Autodesk Inventor part; units mm, degrees
(part 2 of 2)
sketch "Sketch8" plane through (0, 0, 6.35) normal (0, 0, 1) x (1, 0, 0)
  line L0 (104.7603, 19.05) -> (104.7603, 12.7) projected
  line L1 (104.7603, 12.7) -> (59.5313, 12.7) projected
  line L2 (59.5313, 12.7) -> (59.5312, -36.7665) projected
  line L3 (59.5312, -36.7665) -> (65.8813, -36.7665) projected
  line L4 (65.8813, -36.7665) -> (65.8813, -43.1165) projected
  line L5 (65.8813, -43.1165) -> (72.2313, -43.1165) projected
  line L6 (72.2313, -43.1165) -> (72.2313, -36.7665) projected
  line L7 (72.2313, -36.7665) -> (78.5813, -36.7665) projected
  line L8 (78.5813, -36.7665) -> (78.5813, -43.1165) projected
  line L9 (78.5813, -43.1165) -> (84.9313, -43.1165) projected
  line L10 (84.9313, -43.1165) -> (84.9313, -36.7665) projected
  line L11 (84.9313, -36.7665) -> (91.2812, -36.7665) projected
  line L12 (91.2812, -36.7665) -> (91.2812, -43.1165) projected
  line L13 (91.2812, -43.1165) -> (97.6313, -43.1165) projected
  line L14 (97.6313, -43.1165) -> (97.6313, -36.7665) projected
  line L15 (97.6313, -36.7665) -> (103.9813, -36.7665) projected
  line L16 (103.9813, -36.7665) -> (103.9813, -43.1165) projected
  line L17 (103.9813, -43.1165) -> (110.3313, -43.1165) projected
  line L18 (110.3313, -43.1165) -> (110.3313, -36.7665) projected
  line L19 (110.3313, -36.7665) -> (116.6813, -36.7665) projected
  line L20 (116.6813, -36.7665) -> (116.6813, -43.1165) projected
  line L21 (116.6813, -43.1165) -> (123.0313, -43.1165) projected
  line L22 (123.0313, -43.1165) -> (123.0313, -36.7665) projected
  line L23 (123.0313, -36.7665) -> (129.3812, -36.7665) projected
  line L24 (129.3812, -36.7665) -> (129.3812, -43.1165) projected
  line L25 (129.3812, -43.1165) -> (135.7313, -43.1165) projected
  line L26 (135.7313, -43.1165) -> (135.7313, -36.7665) projected
  line L27 (135.7313, -36.7665) -> (142.8603, -36.7665) projected
  line L28 (142.8603, -36.7665) -> (142.8603, -43.1165) projected
  arc A0 (142.8603, -43.1165) -> (143.3542, -41.4448) centre (0, 0) ccw projected
  arc A1 (143.3542, -41.4448) -> (149.3949, -41.0801) centre (144.1598, -4.5833) ccw projected
  arc A2 (149.3949, -41.0801) -> (149.9198, -39.121) centre (0, 0) ccw projected
  arc A3 (149.9198, -39.121) -> (144.8708, -35.7848) centre (127.1377, -68.1106) ccw projected
  arc A4 (144.8708, -35.7848) -> (145.3268, -33.8855) centre (0, 0) ccw projected
  arc A5 (145.3268, -33.8855) -> (151.3401, -33.2051) centre (144.2021, 2.9677) ccw projected
  arc A6 (151.3401, -33.2051) -> (151.7618, -31.2212) centre (0, 0) ccw projected
  arc A7 (151.7618, -31.2212) -> (146.5451, -28.1538) centre (130.5281, -61.3634) ccw projected
  arc A8 (146.5451, -28.1538) -> (146.9011, -26.2332) centre (0, 0) ccw projected
  arc A9 (146.9011, -26.2332) -> (152.8705, -25.239) centre (143.8491, 10.5106) ccw projected
  arc A10 (152.8705, -25.239) -> (153.1878, -23.2358) centre (0, 0) ccw projected
  arc A11 (153.1878, -23.2358) -> (147.8177, -20.4457) centre (133.5607, -54.448) ccw projected
  arc A12 (147.8177, -20.4457) -> (148.0727, -18.509) centre (0, 0) ccw projected
  arc A13 (148.0727, -18.509) -> (153.9819, -17.2038) centre (143.1019, 18.0247) ccw projected
  arc A14 (153.9819, -17.2038) -> (154.1939, -15.1868) centre (0, 0) ccw projected
  arc A15 (154.1939, -15.1868) -> (148.6852, -12.6815) centre (136.2272, -47.3834) ccw projected
  arc A16 (148.6852, -12.6815) -> (148.8384, -10.7342) centre (0, 0) ccw projected
  arc A17 (148.8384, -10.7342) -> (154.6713, -9.1214) centre (141.9624, 25.4894) ccw projected
  arc A18 (154.6713, -9.1214) -> (154.7774, -7.0961) centre (0, 0) ccw projected
  arc A19 (154.7774, -7.0961) -> (149.1451, -4.8825) centre (138.5204, -40.1889) ccw projected
  arc A20 (149.1451, -4.8825) -> (149.1962, -2.9298) centre (0, 0) ccw projected
  arc A21 (149.1962, -2.9298) -> (154.9367, -1.0141) centre (140.4339, 32.8842) ccw projected
  arc A22 (154.9367, -1.0141) -> (154.9367, 1.0141) centre (0, 0) ccw projected
  arc A23 (154.9367, 1.0141) -> (149.1962, 2.9298) centre (140.4339, -32.8842) ccw projected
  arc A24 (149.1962, 2.9298) -> (149.1451, 4.8825) centre (0, 0) ccw projected
  arc A25 (149.1451, 4.8825) -> (154.7774, 7.0961) centre (138.5204, 40.1889) ccw projected
  arc A26 (154.7774, 7.0961) -> (154.6713, 9.1214) centre (0, 0) ccw projected
  arc A27 (154.6713, 9.1214) -> (148.8384, 10.7342) centre (141.9624, -25.4894) ccw projected
  arc A28 (148.8384, 10.7342) -> (148.6852, 12.6815) centre (0, 0) ccw projected
  arc A29 (148.6852, 12.6815) -> (154.1939, 15.1868) centre (136.2272, 47.3834) ccw projected
  arc A30 (154.1939, 15.1868) -> (153.9819, 17.2038) centre (0, 0) ccw projected
  arc A31 (153.9819, 17.2038) -> (148.0727, 18.509) centre (143.1019, -18.0247) ccw projected
  arc A32 (148.0727, 18.509) -> (147.8177, 20.4457) centre (0, 0) ccw projected
  arc A33 (147.8177, 20.4457) -> (153.1878, 23.2358) centre (133.5607, 54.448) ccw projected
  arc A34 (153.1878, 23.2358) -> (152.8705, 25.239) centre (0, 0) ccw projected
  arc A35 (152.8705, 25.239) -> (146.9011, 26.2332) centre (143.8491, -10.5106) ccw projected
  arc A36 (146.9011, 26.2332) -> (146.5451, 28.1538) centre (0, 0) ccw projected
  arc A37 (146.5451, 28.1538) -> (151.7618, 31.2212) centre (130.5281, 61.3634) ccw projected
  arc A38 (151.7618, 31.2212) -> (151.3401, 33.2051) centre (0, 0) ccw projected
  arc A39 (151.3401, 33.2051) -> (145.3268, 33.8855) centre (144.2021, -2.9677) ccw projected
  arc A40 (145.3268, 33.8855) -> (144.8708, 35.7848) centre (0, 0) ccw projected
  arc A41 (144.8708, 35.7848) -> (149.9198, 39.121) centre (127.1377, 68.1106) ccw projected
  arc A42 (149.9198, 39.121) -> (149.3949, 41.0801) centre (0, 0) ccw projected
  arc A43 (149.3949, 41.0801) -> (143.3542, 41.4448) centre (144.1598, 4.5833) ccw projected
  arc A44 (143.3542, 41.4448) -> (142.7994, 43.3177) centre (0, 0) ccw projected
  arc A45 (142.7994, 43.3177) -> (147.6669, 46.9136) centre (123.3988, 74.6712) ccw projected
  arc A46 (147.6669, 46.9136) -> (147.0402, 48.8425) centre (0, 0) ccw projected
  arc A47 (147.0402, 48.8425) -> (140.9887, 48.8906) centre (143.7223, 12.1217) ccw projected
  arc A48 (140.9887, 48.8906) -> (140.3366, 50.7319) centre (0, 0) ccw projected
  arc A49 (140.3366, 50.7319) -> (145.0093, 54.5776) centre (119.3217, 81.027) ccw projected
  arc A50 (145.0093, 54.5776) -> (144.2824, 56.4711) centre (0, 0) ccw projected
  arc A51 (144.2824, 56.4711) -> (138.2367, 56.2024) centre (142.891, 19.627) ccw projected
  arc A52 (138.2367, 56.2024) -> (137.4892, 58.007) centre (0, 0) ccw projected
  arc A53 (137.4892, 58.007) -> (141.9542, 62.092) centre (114.9175, 87.1608) ccw projected
  arc A54 (141.9542, 62.092) -> (141.1292, 63.9448) centre (0, 0) ccw projected
  arc A55 (141.1292, 63.9448) -> (135.1059, 63.3601) centre (141.6679, 27.0784) ccw projected
  arc A56 (135.1059, 63.3601) -> (134.2649, 65.1232) centre (0, 0) ccw projected
  arc A57 (134.2649, 65.1232) -> (138.51, 69.4362) centre (110.1984, 93.0557) ccw projected
  arc A58 (138.51, 69.4362) -> (137.5892, 71.2433) centre (0, 0) ccw projected
  arc A59 (137.5892, 71.2433) -> (131.6047, 70.3442) centre (140.0566, 34.4556) ccw projected
  arc A60 (131.6047, 70.3442) -> (130.6726, 72.0608) centre (0, 0) ccw projected
  arc A61 (130.6726, 72.0608) -> (134.6861, 76.5901) centre (105.1772, 98.6955) ccw projected
  arc A62 (134.6861, 76.5901) -> (133.6721, 78.3466) centre (0, 0) ccw projected
  arc A63 (133.6721, 78.3466) -> (127.7428, 77.1354) centre (138.0614, 41.7384) ccw projected
  arc A64 (127.7428, 77.1354) -> (126.7222, 78.8009) centre (0, 0) ccw projected
  arc A65 (126.7222, 78.8009) -> (130.4931, 83.5341) centre (99.8678, 104.0648) ccw projected
  arc A66 (130.4931, 83.5341) -> (129.3885, 85.235) centre (0, 0) ccw projected
  arc A67 (129.3885, 85.235) -> (123.5308, 83.7153) centre (135.6878, 48.9068) ccw projected
  arc A68 (123.5308, 83.7153) -> (122.4244, 85.3251) centre (0, 0) ccw projected
  arc A69 (122.4244, 85.3251) -> (125.9425, 90.2491) centre (94.2846, 109.1488) ccw projected
  arc A70 (125.9425, 90.2491) -> (124.7504, 91.8899) centre (0, 0) ccw projected
  arc A71 (124.7504, 91.8899) -> (118.9802, 90.0656) centre (132.9422, 55.9411) ccw projected
  arc A72 (118.9802, 90.0656) -> (117.7911, 91.6153) centre (0, 0) ccw projected
  arc A73 (117.7911, 91.6153) -> (121.0466, 96.7167) centre (88.4429, 113.9337) ccw projected
  arc A74 (121.0466, 96.7167) -> (119.7702, 98.2929) centre (0, 0) ccw projected
  arc A75 (119.7702, 98.2929) -> (114.1034, 96.1691) centre (129.8323, 62.8221) ccw projected
  arc A76 (114.1034, 96.1691) -> (112.8349, 97.6545) centre (0, 0) ccw projected
  arc A77 (112.8349, 97.6545) -> (115.8189, 102.9193) centre (82.3589, 118.4063) ccw projected
  arc A78 (115.8189, 102.9193) -> (114.4618, 104.4265) centre (0, 0) ccw projected
  arc A79 (114.4618, 104.4265) -> (108.914, 102.0091) centre (126.3665, 69.5309) ccw projected
  arc A80 (108.914, 102.0091) -> (107.5694, 103.426) centre (0, 0) ccw projected
  arc A81 (107.5694, 103.426) -> (110.2738, 108.8397) centre (76.0491, 122.5544) ccw projected
  arc A82 (110.2738, 108.8397) -> (108.8397, 110.2738) centre (0, 0) ccw projected
  arc A83 (108.8397, 110.2738) -> (103.426, 107.5694) centre (122.5544, 76.0491) ccw projected
  arc A84 (103.426, 107.5694) -> (102.0091, 108.914) centre (0, 0) ccw projected
  arc A85 (102.0091, 108.914) -> (104.4265, 114.4618) centre (69.5309, 126.3665) ccw projected
  arc A86 (104.4265, 114.4618) -> (102.9193, 115.8189) centre (0, 0) ccw projected
  arc A87 (102.9193, 115.8189) -> (97.6545, 112.8349) centre (118.4063, 82.3589) ccw projected
  arc A88 (97.6545, 112.8349) -> (96.1691, 114.1034) centre (0, 0) ccw projected
  arc A89 (96.1691, 114.1034) -> (98.2929, 119.7702) centre (62.8221, 129.8323) ccw projected
  arc A90 (98.2929, 119.7702) -> (96.7167, 121.0466) centre (0, 0) ccw projected
  arc A91 (96.7167, 121.0466) -> (91.6153, 117.7911) centre (113.9337, 88.4429) ccw projected
  arc A92 (91.6153, 117.7911) -> (90.0656, 118.9802) centre (0, 0) ccw projected
  arc A93 (90.0656, 118.9802) -> (91.8899, 124.7504) centre (55.9411, 132.9422) ccw projected
  arc A94 (91.8899, 124.7504) -> (90.2491, 125.9425) centre (0, 0) ccw projected
  arc A95 (90.2491, 125.9425) -> (85.3251, 122.4244) centre (109.1488, 94.2846) ccw projected
  arc A96 (85.3251, 122.4244) -> (83.7153, 123.5308) centre (0, 0) ccw projected
  arc A97 (83.7153, 123.5308) -> (85.235, 129.3885) centre (48.9068, 135.6878) ccw projected
  arc A98 (85.235, 129.3885) -> (83.5341, 130.4931) centre (0, 0) ccw projected
  arc A99 (83.5341, 130.4931) -> (78.8009, 126.7222) centre (104.0648, 99.8678) ccw projected
  arc A100 (78.8009, 126.7222) -> (77.1354, 127.7428) centre (0, 0) ccw projected
  arc A101 (77.1354, 127.7428) -> (78.3466, 133.6721) centre (41.7384, 138.0614) ccw projected
  arc A102 (78.3466, 133.6721) -> (76.5901, 134.6861) centre (0, 0) ccw projected
  arc A103 (76.5901, 134.6861) -> (72.0608, 130.6726) centre (98.6955, 105.1772) ccw projected
  arc A104 (72.0608, 130.6726) -> (70.3442, 131.6047) centre (0, 0) ccw projected
  arc A105 (70.3442, 131.6047) -> (71.2433, 137.5892) centre (34.4556, 140.0566) ccw projected
  arc A106 (71.2433, 137.5892) -> (69.4362, 138.51) centre (0, 0) ccw projected
  arc A107 (69.4362, 138.51) -> (65.1232, 134.2649) centre (93.0557, 110.1984) ccw projected
  arc A108 (65.1232, 134.2649) -> (63.3601, 135.1059) centre (0, 0) ccw projected
  arc A109 (63.3601, 135.1059) -> (63.9448, 141.1292) centre (27.0784, 141.6679) ccw projected
  arc A110 (63.9448, 141.1292) -> (62.092, 141.9542) centre (0, 0) ccw projected
  arc A111 (62.092, 141.9542) -> (58.007, 137.4892) centre (87.1608, 114.9175) ccw projected
  arc A112 (58.007, 137.4892) -> (56.2024, 138.2367) centre (0, 0) ccw projected
  arc A113 (56.2024, 138.2367) -> (56.4711, 144.2824) centre (19.627, 142.891) ccw projected
  arc A114 (56.4711, 144.2824) -> (54.5776, 145.0093) centre (0, 0) ccw projected
  arc A115 (54.5776, 145.0093) -> (50.7319, 140.3366) centre (81.027, 119.3217) ccw projected
  arc A116 (50.7319, 140.3366) -> (48.8906, 140.9887) centre (0, 0) ccw projected
  arc A117 (48.8906, 140.9887) -> (48.8425, 147.0402) centre (12.1217, 143.7223) ccw projected
  arc A118 (48.8425, 147.0402) -> (46.9136, 147.6669) centre (0, 0) ccw projected
  arc A119 (46.9136, 147.6669) -> (43.3177, 142.7994) centre (74.6712, 123.3988) ccw projected
  arc A120 (43.3177, 142.7994) -> (41.4448, 143.3542) centre (0, 0) ccw projected
  arc A121 (41.4448, 143.3542) -> (41.0801, 149.3949) centre (4.5833, 144.1598) ccw projected
  arc A122 (41.0801, 149.3949) -> (39.121, 149.9198) centre (0, 0) ccw projected
  arc A123 (39.121, 149.9198) -> (35.7848, 144.8708) centre (68.1106, 127.1377) ccw projected
  arc A124 (35.7848, 144.8708) -> (33.8855, 145.3268) centre (0, 0) ccw projected
  arc A125 (33.8855, 145.3268) -> (33.2051, 151.3401) centre (-2.9677, 144.2021) ccw projected
  arc A126 (33.2051, 151.3401) -> (31.2212, 151.7618) centre (0, 0) ccw projected
  arc A127 (31.2212, 151.7618) -> (28.1538, 146.5451) centre (61.3634, 130.5281) ccw projected
  arc A128 (28.1538, 146.5451) -> (26.2332, 146.9011) centre (0, 0) ccw projected
  arc A129 (26.2332, 146.9011) -> (25.239, 152.8705) centre (-10.5106, 143.8491) ccw projected
  arc A130 (25.239, 152.8705) -> (23.2358, 153.1878) centre (0, 0) ccw projected
  arc A131 (23.2358, 153.1878) -> (20.4457, 147.8177) centre (54.448, 133.5607) ccw projected
  arc A132 (20.4457, 147.8177) -> (18.509, 148.0727) centre (0, 0) ccw projected
  arc A133 (18.509, 148.0727) -> (17.2038, 153.9819) centre (-18.0247, 143.1019) ccw projected
  arc A134 (17.2038, 153.9819) -> (15.1868, 154.1939) centre (0, 0) ccw projected
  arc A135 (15.1868, 154.1939) -> (12.6815, 148.6852) centre (47.3834, 136.2272) ccw projected
  arc A136 (12.6815, 148.6852) -> (10.7342, 148.8384) centre (0, 0) ccw projected
  arc A137 (10.7342, 148.8384) -> (9.1214, 154.6713) centre (-25.4894, 141.9624) ccw projected
  arc A138 (9.1214, 154.6713) -> (7.0961, 154.7774) centre (0, 0) ccw projected
  arc A139 (7.0961, 154.7774) -> (4.8825, 149.1451) centre (40.1889, 138.5204) ccw projected
  arc A140 (4.8825, 149.1451) -> (2.9298, 149.1962) centre (0, 0) ccw projected
  arc A141 (2.9298, 149.1962) -> (1.0141, 154.9367) centre (-32.8842, 140.4339) ccw projected
  arc A142 (1.0141, 154.9367) -> (-1.0141, 154.9367) centre (0, 0) ccw projected
  arc A143 (-1.0141, 154.9367) -> (-2.9298, 149.1962) centre (32.8842, 140.4339) ccw projected
  arc A144 (-2.9298, 149.1962) -> (-4.8825, 149.1451) centre (0, 0) ccw projected
  arc A145 (-4.8825, 149.1451) -> (-7.0961, 154.7774) centre (-40.1889, 138.5204) ccw projected
  arc A146 (-7.0961, 154.7774) -> (-9.1214, 154.6713) centre (0, 0) ccw projected
  arc A147 (-9.1214, 154.6713) -> (-10.7342, 148.8384) centre (25.4894, 141.9624) ccw projected
  arc A148 (-10.7342, 148.8384) -> (-12.6815, 148.6852) centre (0, 0) ccw projected
  arc A149 (-12.6815, 148.6852) -> (-15.1868, 154.1939) centre (-47.3834, 136.2272) ccw projected
  arc A150 (-15.1868, 154.1939) -> (-17.2038, 153.9819) centre (0, 0) ccw projected
  arc A151 (-17.2038, 153.9819) -> (-18.509, 148.0727) centre (18.0247, 143.1019) ccw projected
  arc A152 (-18.509, 148.0727) -> (-20.4457, 147.8177) centre (0, 0) ccw projected
  arc A153 (-20.4457, 147.8177) -> (-23.2358, 153.1878) centre (-54.448, 133.5607) ccw projected
  arc A154 (-23.2358, 153.1878) -> (-25.239, 152.8705) centre (0, 0) ccw projected
  arc A155 (-25.239, 152.8705) -> (-26.2332, 146.9011) centre (10.5106, 143.8491) ccw projected
  arc A156 (-26.2332, 146.9011) -> (-28.1538, 146.5451) centre (0, 0) ccw projected
  arc A157 (-28.1538, 146.5451) -> (-31.2212, 151.7618) centre (-61.3634, 130.5281) ccw projected
  arc A158 (-31.2212, 151.7618) -> (-33.2051, 151.3401) centre (0, 0) ccw projected
  arc A159 (-33.2051, 151.3401) -> (-33.8855, 145.3268) centre (2.9677, 144.2021) ccw projected
  arc A160 (-33.8855, 145.3268) -> (-35.7848, 144.8708) centre (0, 0) ccw projected
  arc A161 (-35.7848, 144.8708) -> (-39.121, 149.9198) centre (-68.1106, 127.1377) ccw projected
  arc A162 (-39.121, 149.9198) -> (-41.0801, 149.3949) centre (0, 0) ccw projected
  arc A163 (-41.0801, 149.3949) -> (-41.4448, 143.3542) centre (-4.5833, 144.1598) ccw projected
  arc A164 (-41.4448, 143.3542) -> (-43.3177, 142.7994) centre (0, 0) ccw projected
  arc A165 (-43.3177, 142.7994) -> (-46.9136, 147.6669) centre (-74.6712, 123.3988) ccw projected
  arc A166 (-46.9136, 147.6669) -> (-48.8425, 147.0402) centre (0, 0) ccw projected
  arc A167 (-48.8425, 147.0402) -> (-48.8906, 140.9887) centre (-12.1217, 143.7223) ccw projected
  arc A168 (-48.8906, 140.9887) -> (-50.7319, 140.3366) centre (0, 0) ccw projected
  arc A169 (-50.7319, 140.3366) -> (-54.5776, 145.0093) centre (-81.027, 119.3217) ccw projected
  arc A170 (-54.5776, 145.0093) -> (-56.4711, 144.2824) centre (0, 0) ccw projected
  arc A171 (-56.4711, 144.2824) -> (-56.2024, 138.2367) centre (-19.627, 142.891) ccw projected
  arc A172 (-56.2024, 138.2367) -> (-58.007, 137.4892) centre (0, 0) ccw projected
  arc A173 (-58.007, 137.4892) -> (-62.092, 141.9542) centre (-87.1608, 114.9175) ccw projected
  arc A174 (-62.092, 141.9542) -> (-63.9448, 141.1292) centre (0, 0) ccw projected
  arc A175 (-63.9448, 141.1292) -> (-63.3601, 135.1059) centre (-27.0784, 141.6679) ccw projected
  arc A176 (-63.3601, 135.1059) -> (-65.1232, 134.2649) centre (0, 0) ccw projected
  arc A177 (-65.1232, 134.2649) -> (-69.4362, 138.51) centre (-93.0557, 110.1984) ccw projected
  arc A178 (-69.4362, 138.51) -> (-71.2433, 137.5892) centre (0, 0) ccw projected
  arc A179 (-71.2433, 137.5892) -> (-70.3442, 131.6047) centre (-34.4556, 140.0566) ccw projected
  arc A180 (-70.3442, 131.6047) -> (-72.0608, 130.6726) centre (0, 0) ccw projected
  arc A181 (-72.0608, 130.6726) -> (-76.5901, 134.6861) centre (-98.6955, 105.1772) ccw projected
  arc A182 (-76.5901, 134.6861) -> (-78.3466, 133.6721) centre (0, 0) ccw projected
  arc A183 (-78.3466, 133.6721) -> (-77.1354, 127.7428) centre (-41.7384, 138.0614) ccw projected
  arc A184 (-77.1354, 127.7428) -> (-78.8009, 126.7222) centre (0, 0) ccw projected
  arc A185 (-78.8009, 126.7222) -> (-83.5341, 130.4931) centre (-104.0648, 99.8678) ccw projected
  arc A186 (-83.5341, 130.4931) -> (-85.235, 129.3885) centre (0, 0) ccw projected
  arc A187 (-85.235, 129.3885) -> (-83.7153, 123.5308) centre (-48.9068, 135.6878) ccw projected
  arc A188 (-83.7153, 123.5308) -> (-85.3251, 122.4244) centre (0, 0) ccw projected
  arc A189 (-85.3251, 122.4244) -> (-90.2491, 125.9425) centre (-109.1488, 94.2846) ccw projected
  arc A190 (-90.2491, 125.9425) -> (-91.8899, 124.7504) centre (0, 0) ccw projected
  arc A191 (-91.8899, 124.7504) -> (-90.0656, 118.9802) centre (-55.9411, 132.9422) ccw projected
  arc A192 (-90.0656, 118.9802) -> (-91.6153, 117.7911) centre (0, 0) ccw projected
  arc A193 (-91.6153, 117.7911) -> (-96.7167, 121.0466) centre (-113.9337, 88.4429) ccw projected
  arc A194 (-96.7167, 121.0466) -> (-98.2929, 119.7702) centre (0, 0) ccw projected
  arc A195 (-98.2929, 119.7702) -> (-96.1691, 114.1034) centre (-62.8221, 129.8323) ccw projected
  arc A196 (-96.1691, 114.1034) -> (-97.6545, 112.8349) centre (0, 0) ccw projected
  arc A197 (-97.6545, 112.8349) -> (-102.9193, 115.8189) centre (-118.4063, 82.3589) ccw projected
  arc A198 (-102.9193, 115.8189) -> (-104.4265, 114.4618) centre (0, 0) ccw projected
  arc A199 (-104.4265, 114.4618) -> (-102.0091, 108.914) centre (-69.5309, 126.3665) ccw projected
  arc A200 (-102.0091, 108.914) -> (-103.426, 107.5694) centre (0, 0) ccw projected
  arc A201 (-103.426, 107.5694) -> (-108.8397, 110.2738) centre (-122.5544, 76.0491) ccw projected
  arc A202 (-108.8397, 110.2738) -> (-110.2738, 108.8397) centre (0, 0) ccw projected
  arc A203 (-110.2738, 108.8397) -> (-107.5694, 103.426) centre (-76.0491, 122.5544) ccw projected
  arc A204 (-107.5694, 103.426) -> (-108.914, 102.0091) centre (0, 0) ccw projected
  arc A205 (-108.914, 102.0091) -> (-114.4618, 104.4265) centre (-126.3665, 69.5309) ccw projected
  arc A206 (-114.4618, 104.4265) -> (-115.8189, 102.9193) centre (0, 0) ccw projected
  arc A207 (-115.8189, 102.9193) -> (-112.8349, 97.6545) centre (-82.3589, 118.4063) ccw projected
  arc A208 (-112.8349, 97.6545) -> (-114.1034, 96.1691) centre (0, 0) ccw projected
  arc A209 (-114.1034, 96.1691) -> (-119.7702, 98.2929) centre (-129.8323, 62.8221) ccw projected
  arc A210 (-119.7702, 98.2929) -> (-121.0466, 96.7167) centre (0, 0) ccw projected
  arc A211 (-121.0466, 96.7167) -> (-117.7911, 91.6153) centre (-88.4429, 113.9337) ccw projected
  arc A212 (-117.7911, 91.6153) -> (-118.9802, 90.0656) centre (0, 0) ccw projected
  arc A213 (-118.9802, 90.0656) -> (-124.7504, 91.8899) centre (-132.9422, 55.9411) ccw projected
  arc A214 (-124.7504, 91.8899) -> (-125.9425, 90.2491) centre (0, 0) ccw projected
  arc A215 (-125.9425, 90.2491) -> (-122.4244, 85.3251) centre (-94.2846, 109.1488) ccw projected
  arc A216 (-122.4244, 85.3251) -> (-123.5308, 83.7153) centre (0, 0) ccw projected
  arc A217 (-123.5308, 83.7153) -> (-129.3885, 85.235) centre (-135.6878, 48.9068) ccw projected
  arc A218 (-129.3885, 85.235) -> (-130.4931, 83.5341) centre (0, 0) ccw projected
  arc A219 (-130.4931, 83.5341) -> (-126.7222, 78.8009) centre (-99.8678, 104.0648) ccw projected
  arc A220 (-126.7222, 78.8009) -> (-127.7428, 77.1354) centre (0, 0) ccw projected
  arc A221 (-127.7428, 77.1354) -> (-133.6721, 78.3466) centre (-138.0614, 41.7384) ccw projected
  arc A222 (-133.6721, 78.3466) -> (-134.6861, 76.5901) centre (0, 0) ccw projected
  arc A223 (-134.6861, 76.5901) -> (-130.6726, 72.0608) centre (-105.1772, 98.6955) ccw projected
  arc A224 (-130.6726, 72.0608) -> (-131.6047, 70.3442) centre (0, 0) ccw projected
  arc A225 (-131.6047, 70.3442) -> (-137.5892, 71.2433) centre (-140.0566, 34.4556) ccw projected
  arc A226 (-137.5892, 71.2433) -> (-138.51, 69.4362) centre (0, 0) ccw projected
  arc A227 (-138.51, 69.4362) -> (-134.2649, 65.1232) centre (-110.1984, 93.0557) ccw projected
  arc A228 (-134.2649, 65.1232) -> (-135.1059, 63.3601) centre (0, 0) ccw projected
  arc A229 (-135.1059, 63.3601) -> (-141.1292, 63.9448) centre (-141.6679, 27.0784) ccw projected
  arc A230 (-141.1292, 63.9448) -> (-141.9542, 62.092) centre (0, 0) ccw projected
  arc A231 (-141.9542, 62.092) -> (-137.4892, 58.007) centre (-114.9175, 87.1608) ccw projected
  arc A232 (-137.4892, 58.007) -> (-138.2367, 56.2024) centre (0, 0) ccw projected
  arc A233 (-138.2367, 56.2024) -> (-144.2824, 56.4711) centre (-142.891, 19.627) ccw projected
  arc A234 (-144.2824, 56.4711) -> (-145.0093, 54.5776) centre (0, 0) ccw projected
  arc A235 (-145.0093, 54.5776) -> (-140.3366, 50.7319) centre (-119.3217, 81.027) ccw projected
  arc A236 (-140.3366, 50.7319) -> (-140.9887, 48.8906) centre (0, 0) ccw projected
  arc A237 (-140.9887, 48.8906) -> (-147.0402, 48.8425) centre (-143.7223, 12.1217) ccw projected
  arc A238 (-147.0402, 48.8425) -> (-147.6669, 46.9136) centre (0, 0) ccw projected
  arc A239 (-147.6669, 46.9136) -> (-142.7994, 43.3177) centre (-123.3988, 74.6712) ccw projected
  arc A240 (-142.7994, 43.3177) -> (-143.3542, 41.4448) centre (0, 0) ccw projected
  arc A241 (-143.3542, 41.4448) -> (-149.3949, 41.0801) centre (-144.1598, 4.5833) ccw projected
  arc A242 (-149.3949, 41.0801) -> (-149.9198, 39.121) centre (0, 0) ccw projected
  arc A243 (-149.9198, 39.121) -> (-144.8708, 35.7848) centre (-127.1377, 68.1106) ccw projected
  arc A244 (-144.8708, 35.7848) -> (-145.3268, 33.8855) centre (0, 0) ccw projected
  arc A245 (-145.3268, 33.8855) -> (-151.3401, 33.2051) centre (-144.2021, -2.9677) ccw projected
  arc A246 (-151.3401, 33.2051) -> (-151.7618, 31.2212) centre (0, 0) ccw projected
  arc A247 (-151.7618, 31.2212) -> (-146.5451, 28.1538) centre (-130.5281, 61.3634) ccw projected
  arc A248 (-146.5451, 28.1538) -> (-146.9011, 26.2332) centre (0, 0) ccw projected
  arc A249 (-146.9011, 26.2332) -> (-152.8705, 25.239) centre (-143.8491, -10.5106) ccw projected
  arc A250 (-152.8705, 25.239) -> (-153.1878, 23.2358) centre (0, 0) ccw projected
  arc A251 (-153.1878, 23.2358) -> (-147.8177, 20.4457) centre (-133.5607, 54.448) ccw projected
  arc A252 (-147.8177, 20.4457) -> (-148.0727, 18.509) centre (0, 0) ccw projected
  arc A253 (-148.0727, 18.509) -> (-153.9819, 17.2038) centre (-143.1019, -18.0247) ccw projected
  arc A254 (-153.9819, 17.2038) -> (-154.1939, 15.1868) centre (0, 0) ccw projected
  arc A255 (-154.1939, 15.1868) -> (-148.6852, 12.6815) centre (-136.2272, 47.3834) ccw projected
  arc A256 (-148.6852, 12.6815) -> (-148.8384, 10.7342) centre (0, 0) ccw projected
  arc A257 (-148.8384, 10.7342) -> (-154.6713, 9.1214) centre (-141.9624, -25.4894) ccw projected
  arc A258 (-154.6713, 9.1214) -> (-154.7774, 7.0961) centre (0, 0) ccw projected
  arc A259 (-154.7774, 7.0961) -> (-149.1451, 4.8825) centre (-138.5204, 40.1889) ccw projected
  arc A260 (-149.1451, 4.8825) -> (-149.1962, 2.9298) centre (0, 0) ccw projected
  arc A261 (-149.1962, 2.9298) -> (-154.9367, 1.0141) centre (-140.4339, -32.8842) ccw projected
  arc A262 (-154.9367, 1.0141) -> (-154.9367, -1.0141) centre (0, 0) ccw projected
  arc A263 (-154.9367, -1.0141) -> (-149.1962, -2.9298) centre (-140.4339, 32.8842) ccw projected
  arc A264 (-149.1962, -2.9298) -> (-149.1451, -4.8825) centre (0, 0) ccw projected
  arc A265 (-149.1451, -4.8825) -> (-154.7774, -7.0961) centre (-138.5204, -40.1889) ccw projected
  arc A266 (-154.7774, -7.0961) -> (-154.6713, -9.1214) centre (0, 0) ccw projected
  arc A267 (-154.6713, -9.1214) -> (-148.8384, -10.7342) centre (-141.9624, 25.4894) ccw projected
  arc A268 (-148.8384, -10.7342) -> (-148.6852, -12.6815) centre (0, 0) ccw projected
  arc A269 (-148.6852, -12.6815) -> (-154.1939, -15.1868) centre (-136.2272, -47.3834) ccw projected
  arc A270 (-154.1939, -15.1868) -> (-153.9819, -17.2038) centre (0, 0) ccw projected
  arc A271 (-153.9819, -17.2038) -> (-148.0727, -18.509) centre (-143.1019, 18.0247) ccw projected
  arc A272 (-148.0727, -18.509) -> (-147.8177, -20.4457) centre (0, 0) ccw projected
  arc A273 (-147.8177, -20.4457) -> (-153.1878, -23.2358) centre (-133.5607, -54.448) ccw projected
  arc A274 (-153.1878, -23.2358) -> (-152.8705, -25.239) centre (0, 0) ccw projected
  arc A275 (-152.8705, -25.239) -> (-146.9011, -26.2332) centre (-143.8491, 10.5106) ccw projected
  arc A276 (-146.9011, -26.2332) -> (-146.5451, -28.1538) centre (0, 0) ccw projected
  arc A277 (-146.5451, -28.1538) -> (-151.7618, -31.2212) centre (-130.5281, -61.3634) ccw projected
  arc A278 (-151.7618, -31.2212) -> (-151.3401, -33.2051) centre (0, 0) ccw projected
  arc A279 (-151.3401, -33.2051) -> (-145.3268, -33.8855) centre (-144.2021, 2.9677) ccw projected
  arc A280 (-145.3268, -33.8855) -> (-144.8708, -35.7848) centre (0, 0) ccw projected
  arc A281 (-144.8708, -35.7848) -> (-149.9198, -39.121) centre (-127.1377, -68.1106) ccw projected
  arc A282 (-149.9198, -39.121) -> (-149.3949, -41.0801) centre (0, 0) ccw projected
  arc A283 (-149.3949, -41.0801) -> (-143.3542, -41.4448) centre (-144.1598, -4.5833) ccw projected
  arc A284 (-143.3542, -41.4448) -> (-142.8603, -43.1165) centre (0, 0) ccw projected
  line L29 (-142.8603, -43.1165) -> (-142.8603, -36.7665) projected
  line L30 (-142.8603, -36.7665) -> (-135.7313, -36.7665) projected
  line L31 (-135.7313, -36.7665) -> (-135.7313, -43.1165) projected
  line L32 (-135.7313, -43.1165) -> (-129.3812, -43.1165) projected
  line L33 (-129.3812, -43.1165) -> (-129.3812, -36.7665) projected
  line L34 (-129.3812, -36.7665) -> (-123.0313, -36.7665) projected
  line L35 (-123.0313, -36.7665) -> (-123.0313, -43.1165) projected
  line L36 (-123.0313, -43.1165) -> (-116.6813, -43.1165) projected
  line L37 (-116.6813, -43.1165) -> (-116.6813, -36.7665) projected
  line L38 (-116.6813, -36.7665) -> (-110.3313, -36.7665) projected
  line L39 (-110.3313, -36.7665) -> (-110.3313, -43.1165) projected
  line L40 (-110.3313, -43.1165) -> (-103.9813, -43.1165) projected
  line L41 (-103.9813, -43.1165) -> (-103.9813, -36.7665) projected
  line L42 (-103.9813, -36.7665) -> (-97.6313, -36.7665) projected
  line L43 (-97.6313, -36.7665) -> (-97.6313, -43.1165) projected
  line L44 (-97.6313, -43.1165) -> (-91.2812, -43.1165) projected
  line L45 (-91.2812, -43.1165) -> (-91.2812, -36.7665) projected
  line L46 (-91.2812, -36.7665) -> (-84.9313, -36.7665) projected
  line L47 (-84.9313, -36.7665) -> (-84.9313, -43.1165) projected
  line L48 (-84.9313, -43.1165) -> (-78.5813, -43.1165) projected
  line L49 (-78.5813, -43.1165) -> (-78.5813, -36.7665) projected
  line L50 (-78.5813, -36.7665) -> (-72.2313, -36.7665) projected
  line L51 (-72.2313, -36.7665) -> (-72.2313, -43.1165) projected
  line L52 (-72.2313, -43.1165) -> (-65.8813, -43.1165) projected
  line L53 (-65.8813, -43.1165) -> (-65.8813, -36.7665) projected
  line L54 (-65.8813, -36.7665) -> (-59.5312, -36.7665) projected
  line L55 (-59.5312, -36.7665) -> (-59.5313, 12.7) projected
  line L56 (-59.5313, 12.7) -> (-104.7603, 12.7) projected
  line L57 (-104.7603, 12.7) -> (-104.7603, 19.05) projected
  line L58 (-104.7603, 19.05) -> (-59.5313, 19.05) projected
  line L59 (-59.5313, 19.05) -> (-59.5312, 44.45) projected
  line L60 (-59.5312, 44.45) -> (-38.1, 44.45) projected
  line L61 (-38.1, 44.45) -> (-38.1, 133.985) projected
  arc A285 (38.1, 133.985) -> (-38.1, 133.985) centre (0, -0.4192) ccw projected
  line L62 (38.1, 133.985) -> (38.1, 44.45) projected
  line L63 (38.1, 44.45) -> (59.5312, 44.45) projected
  line L64 (59.5312, 44.45) -> (59.5313, 19.05) projected
  line L65 (59.5313, 19.05) -> (104.7603, 19.05) projected
  line L66 (-210.1511, -0.4192) -> (214.329, -0.4192)
  constraints: 2 end point
equation "\"d0\" = da_da"
equation "\"d1\" = da_b"
equation "\"d3\" = da_dw"
equation "\"d15\" = da_aw"
equation "\"d19\" = da_aw"
equation "\"da_da\" = 309.88"
equation "\"da_b\" = 6.35"
equation "\"da_dw\" = 304.8"
equation "\"da_aw\" = 176.53"
body "Solid1"
body "Srf1"
